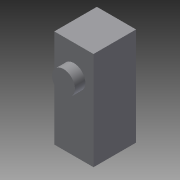
# Autodesk Inventor part: Servo
Saved by Autodesk Inventor 2013 (Build 170138000, 138)
## iProperties
Created: 2013-04-20
Part Number: Servo
Material: Generic
Document SubType Name: Modeling
Designer: fuji
Density: 1 g/cm^3
Author: fuji
Autodesk Inventor part; units mm, degrees
ref_plane "YZ Plane" through (0, 0, 0) normal (1, 0, 0) x (0, 1, 0)
ref_plane "XZ Plane" through (0, 0, 0) normal (0, 1, 0) x (-1, 0, 0)
ref_plane "XY Plane" through (0, 0, 0) normal (0, 0, 1) x (1, 0, 0)
sketch "Sketch1" plane through (0, 0, 0) normal (0, 0, 1) x (1, 0, 0)
  line L0 (0, 0) -> (12, 0)
  line L1 (12, 0) -> (12, 30)
  line L2 (12, 30) -> (0, 30)
  line L3 (0, 30) -> (0, 0)
  dimension "d0" = 12
  dimension "d1" = 30
  constraints: 8 end point, 2 parallel, 1 horizontal, 1 perpendicular
  measures "d0" distance of L2.end L1.end
  measures "d1" distance of L1.end L0.end
extrude "Extrusion1" add sketch "Sketch1" along normal blind 13.0302
sketch "Sketch2" plane through (0, 0, 13.0302) normal (0, 0, 1) x (1, 0, 0)
  line L0 (12, 30) -> (0, 30) projected
  line L1 (0, 30) -> (0, 0) projected
  circle A0 centre (6, 21.11) radius 3.5052
  dimension "d4" = 6
  dimension "d5" = 8.89
  dimension "d8" = 7.0104
  constraints: 1 centre point
  measures "d4" distance from line of L1 A0.centre
  measures "d5" distance from line of A0.centre L0
  measures "d8" diameter of A0
extrude "Extrusion2" add sketch "Sketch2" along normal blind 3.175
equation "\"d0\" = servoWidth"
equation "\"d1\" = servoLength"
equation "\"d2\" = servoHeight"
equation "\"d4\" = 0.5 * servoWidth"
equation "\"d5\" = hornOffset"
equation "\"d8\" = hornCenter"
equation "\"d6\" = thick"
equation "\"servoLength\" = 30"
equation "\"servoWidth\" = 12"
equation "\"hornCenter\" = 7.0104"
equation "\"hornDia\" = 13.1572"
equation "\"hornHole\" = 1.524"
equation "\"hornOffset\" = 8.89"
equation "\"servoHeight\" = 13.0302"
equation "\"thick\" = 3.175"
body "Solid1"
